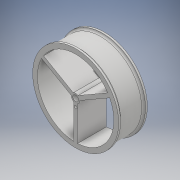
# Autodesk Inventor part: Wheel
Saved by Autodesk Inventor 2018 (Build 220112000, 112)
## iProperties
Created: 2020-02-11
Part Number: Wheel
Material: Типовые
Document SubType Name: Modeling
Designer: cosko
Density: 1 g/cm^3
Appearance: По умолчанию
Author: cosko
Autodesk Inventor part; units mm, degrees
ref_plane "YZ Plane" through (0, 0, 0) normal (1, 0, 0) x (0, 1, 0)
ref_plane "XZ Plane" through (0, 0, 0) normal (0, 1, 0) x (-1, 0, 0)
ref_plane "XY Plane" through (0, 0, 0) normal (0, 0, 1) x (1, 0, 0)
sketch "Эскиз1" plane through (0, 0, 0) normal (0, 0, 1) x (1, 0, 0)
  line L0 (0, 0) -> (40, 0)
  line L1 (0, 0) -> (0, 10)
  line L2 (40, 0) -> (40, -15) construction
  line L3 (40, -15) -> (45, -15)
  line L4 (45, 15) -> (40, 15)
  line L5 (40, 15) -> (40, -15)
  line L6 (40, 15) -> (40, 13) construction
  line L7 (40, 13) -> (45, 13) construction
  line L8 (40, -15) -> (40, -13) construction
  line L9 (40, -13) -> (45, -13) construction
  line L10 (45, -13) -> (45, -11) construction
  line L11 (45, -11) -> (45, -9) construction
  arc A0 (43, -11) -> (45, -13) centre (45, -11) ccw
  arc A1 (45, 13) -> (43, 11) centre (45, 11) ccw
  line L12 (43, 11) -> (43, -11)
  line L13 (45, -15) -> (45, -13)
  line L14 (45, 13) -> (45, 15)
  dimension "d0" = 40
  dimension "d1" = 10
  dimension "d2" = 15
  dimension "d3" = 5
  dimension "d4" = 30
  dimension "d5" = 2
  dimension "d6" = 2
  constraints: 30 end point, 6 perpendicular, 4 point on circle, 3 parallel, 2 centre point, 2 horizontal, 2 point on line, 2 vertical, 1 coincident
  measures "d0" distance of L0.start L0.end
  measures "d1" distance of L0.start L1.end
  measures "d2" distance of L0.end L2.end
  measures "d3" distance of L4.end L4.start
  measures "d4" distance of L4.start L3.end
  measures "d5" distance of L4.end L6.end
  measures "d6" distance of L2.end L8.end
revolve "Вращение1" add sketch "Эскиз1" angle 360 about axis through (0, 0, 0) along (0, 1, 0)
sketch "Эскиз7" plane through (0, 15, 0) normal (0, 1, 0) x (1, 0, 0)
  circle A0 centre (0, 0) radius 11
  dimension "d29" = 22
  constraints: 1 centre point, 1 coincident
  measures "d29" diameter of A0
extrude "Выдавливание5" add sketch "Эскиз7" against normal blind 3
sketch "Эскиз8" plane through (0, 15, 0) normal (0, 1, 0) x (1, 0, 0)
  circle A0 centre (0, 0) radius 3
  circle A1 centre (0, 0) radius 4.5
  dimension "d32" = 6
  dimension "d33" = 9
  constraints: 2 centre point, 2 coincident
  measures "d32" diameter of A0
  measures "d33" diameter of A1
extrude "Выдавливание6" cut sketch "Эскиз8" against normal blind 3 contours A0
extrude "Выдавливание7" add sketch "Эскиз8" against normal up to surface (30 mm away)
sketch "Эскиз10" plane through (0, 15, 0) normal (0, 1, 0) x (1, 0, 0)
  line L0 (0, 0) -> (8, 0) construction
  circle A0 centre (8, 0) radius 1.5
  circle A1 centre (0, 0) radius 3 construction
  circle A2 centre (0, 8) radius 1.5
  circle A3 centre (-8, 0) radius 1.5
  circle A4 centre (0, -8) radius 1.5
  dimension "d38" = 8
  dimension "d39" = 3
  dimension "d42" = 360
  constraints: 5 centre point, 2 coincident, 2 end point, 1 horizontal, 9 other
  measures "d38" distance of L0.start L0.end
  measures "d39" diameter of A0
extrude "Выдавливание8" cut sketch "Эскиз10" against normal blind 3
sketch "Эскиз11" plane through (0, -15, 0) normal (0, -1, 0) x (1, 0, 0)
  circle A0 centre (0, 0) radius 3 projected
  circle A1 centre (0, 0) radius 4.5 projected
  circle A2 centre (0, 0) radius 45 projected
  circle A3 centre (0, 0) radius 40 projected
  line L0 (0, -4.5) -> (0, -40) construction
  circle A4 centre (0, 0) radius 40 construction
  line L1 (-2, -39.95) -> (-2, -4.0311)
  line L2 (2, -4.0311) -> (2, -39.95)
  line L3 (1.8638, -39.9566) -> (-1.9134, -4.073) construction
  line L4 (-1.8638, -39.9566) -> (1.9134, -4.073) construction
  circle A5 centre (0, -8) radius 1.5 projected
  arc A6 (-2, -39.95) -> (2, -39.95) centre (0, 0) ccw
  arc A7 (-2, -4.0311) -> (1.9134, -4.073) centre (0, 0) ccw
  point P0 (0, -22.25)
  constraints: 16 point on circle, 10 end point, 2 centre point, 2 point on line, 1 midpoint, 1 parallel, 1 vertical
extrude "Выдавливание9" add sketch "Эскиз11" against normal up to surface (30 mm away) contours A1 L2 A3 L1 | A5 picked at (0.0603, -29.826)
pattern_circular "Круговой массив1" count 3 over 360 about axis through (0, 15, 0) along (0, -1, 0) of "Выдавливание9"
sketch "Эскиз12" plane through (0, 15, 0) normal (0, 1, 0) x (1, 0, 0)
  circle A0 centre (8, 0) radius 1.5 projected
  circle A1 centre (0, 0) radius 3 projected
  circle A2 centre (8, 0) radius 1.5
  circle A3 centre (0, 8) radius 1.5
  circle A4 centre (-8, 0) radius 1.5
  circle A5 centre (0, -8) radius 1.5
  dimension "d55" = 360
  constraints: 4 centre point, 1 coincident, 1 concentric, 9 other
extrude "Выдавливание10" cut sketch "Эскиз12" against normal up to next contours A3
